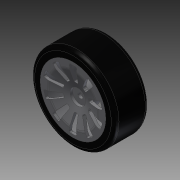
# Autodesk Inventor part: ModellingWheel_65mm
Saved by Autodesk Inventor 2014 SP1 (Build 180222100, 222)
## iProperties
Created: 2015-04-19
Part Number: ModellingWheel_65mm
Material: Rubber
Document SubType Name: Modeling
Designer: david
Density: 0.93 g/cm^3
Appearance: Rubber - Black - Version 1.1
Mass: 44.3361 g
Surface Area: 161.393 cm^2
Volume: 47.6732 cm^3
Author: david
Autodesk Inventor part; units mm, degrees
ref_plane "YZ Plane" through (0, 0, 0) normal (1, 0, 0) x (0, 1, 0)
ref_plane "XZ Plane" through (0, 0, 0) normal (0, 1, 0) x (-1, 0, 0)
ref_plane "XY Plane" through (0, 0, 0) normal (0, 0, 1) x (1, 0, 0)
sketch "Sketch1" plane through (0, 0, 0) normal (1, 0, 0) x (0, 1, 0)
  line L0 (0, 2) -> (0, 6)
  line L1 (0, 0) -> (0, -6.7762) construction
  line L2 (0, 2) -> (6.5, 2)
  line L3 (6.5, 2) -> (6.5, 9)
  line L4 (0, 0) -> (28.6637, 0) construction
  line L5 (6.5, 9) -> (0, 9)
  line L6 (0, 9) -> (-3.75, 19.25)
  line L7 (-3.75, 19.25) -> (-3.75, 23.25)
  line L8 (-3.75, 23.25) -> (20.5, 23.25)
  line L9 (20.5, 23.25) -> (20.5, 25.25)
  line L10 (20.5, 25.25) -> (-5.75, 25.25)
  line L11 (-5.75, 25.25) -> (-5.75, 19.25)
  line L12 (0, 6) -> (-2, 6)
  line L13 (-2, 6) -> (-5.75, 19.25)
  line L14 (-5.75, 19.25) -> (0.5106, 19.25) construction
  dimension "d0" = 4
  dimension "d1" = 2
  dimension "d2" = 6.5
  dimension "d3" = 9
  dimension "d4" = 23.25
  dimension "d5" = 2
  dimension "d6" = 14
  dimension "d7" = 26.25
  dimension "d8" = 2
  dimension "d9" = 2
  dimension "d10" = 6
  constraints: 30 end point, 9 perpendicular, 2 collinear, 2 parallel, 2 point on line, 1 vertical
  measures "d0" distance of L0.start L0.end
  measures "d1" distance of L1.start L0.start
  measures "d2" distance of L0.start L2.end
  measures "d3" distance from line of L4 L3.end
  measures "d4" distance between parallel lines of L4 L8
  measures "d5" distance between parallel lines of L8 L10
  measures "d6" distance between parallel lines of L9 L3
  measures "d7" distance between parallel lines of L9 L11
  measures "d8" distance between parallel lines of L11 L7
  measures "d9" distance of L0.end L12.end
  measures "d10" distance of L10.end L11.end
revolve "Revolution1" add sketch "Sketch1" angle 360 about axis through (0, 0, 0) along (0, 1, 0)
sketch "Sketch2" plane through (0, 20.5, 0) normal (0, 1, 0) x (1, 0, 0)
  circle A0 centre (0, 0) radius 25.25 projected
  circle A1 centre (0, 0) radius 32.5
  dimension "d12" = 65
  constraints: 1 centre point, 1 coincident
  measures "d12" diameter of A1
extrude "Extrusion1" add sketch "Sketch2" against normal up to surface (26.25 mm away) separate body
fillet "Fillet1" radius 3 2 edges at (-32.5, -5.75, 0) (-32.5, 20.5, 0)
sketch "Sketch3" plane through (0, 6.5, 0) normal (0, 1, 0) x (1, 0, 0)
  circle A0 centre (0, 0) radius 2 projected
  circle A1 centre (0, 0) radius 9 projected
  line L0 (6.9282, 0) -> (3.4641, -6)
  line L1 (3.4641, -6) -> (-3.4641, -6)
  line L2 (-3.4641, -6) -> (-6.9282, 0)
  line L3 (-6.9282, 0) -> (-3.4641, 6)
  line L4 (-3.4641, 6) -> (3.4641, 6)
  line L5 (3.4641, 6) -> (6.9282, 0)
  line L6 (0, 0) -> (12.5028, 0) construction
  dimension "d16" = 12
  constraints: 14 end point, 1 coincident, 1 horizontal, 1 point on line, 13 other
  measures "d16" distance between parallel lines of L0 L3
extrude "Extrusion2" cut sketch "Sketch3" against normal blind 4.5 contours L0 L1 L2 L3 L4 L5 bodies 1
sketch "Sketch4" plane through (0, -5.75, 0) normal (0, -1, 0) x (1, 0, 0)
  circle A0 centre (0, 0) radius 25.25 projected
  circle A1 centre (0, 0) radius 19.25 projected
  line L0 (-1.878, 23) -> (1.878, 23)
  line L1 (2.8714, 21.8854) -> (1.6022, 10.8854)
  line L2 (0.6087, 10) -> (-0.6087, 10)
  line L3 (-1.6022, 10.8854) -> (-2.8714, 21.8854)
  line L4 (0, 0) -> (0, 46.8233) construction
  circle A2 centre (0, 0) radius 19.25 construction
  circle A3 centre (0, 0) radius 6 construction
  circle A4 centre (0, 0) radius 25.25 construction
  circle A5 centre (0, 0) radius 19.25 construction
  circle A6 centre (0, 0) radius 19.25 construction
  circle A7 centre (0, 0) radius 25.25 construction
  circle A8 centre (0, 0) radius 29.5 construction
  circle A9 centre (0, 0) radius 25.25 construction
  arc A10 (-1.6022, 10.8854) -> (-0.6087, 10) centre (-0.6087, 11) ccw
  arc A11 (0.6087, 10) -> (1.6022, 10.8854) centre (0.6087, 11) ccw
  arc A12 (-1.878, 23) -> (-2.8714, 21.8854) centre (-1.878, 22) ccw
  arc A13 (2.8714, 21.8854) -> (1.878, 23) centre (1.878, 22) ccw
  line L5 (11.9997, 19.7112) -> (15.0384, 17.5035)
  line L6 (15.1869, 16.0179) -> (7.6944, 7.8647)
  line L7 (6.3703, 7.7324) -> (5.3854, 8.448)
  line L8 (5.1021, 9.7482) -> (10.5409, 19.3934)
  arc A14 (5.1021, 9.7482) -> (5.3854, 8.448) centre (5.9731, 9.257) ccw
  arc A15 (6.3703, 7.7324) -> (7.6944, 7.8647) centre (6.9581, 8.5414) ccw
  arc A16 (11.9997, 19.7112) -> (10.5409, 19.3934) centre (11.412, 18.9022) ccw
  arc A17 (15.1869, 16.0179) -> (15.0384, 17.5035) centre (14.4506, 16.6945) ccw
  line L9 (21.294, 8.8935) -> (22.4546, 5.3213)
  line L10 (21.7015, 4.0321) -> (10.8477, 1.84)
  line L11 (9.6987, 2.5112) -> (9.3225, 3.6691)
  line L12 (9.8575, 4.8875) -> (19.9269, 9.4938)
  arc A18 (9.8575, 4.8875) -> (9.3225, 3.6691) centre (10.2735, 3.9781) ccw
  arc A19 (9.6987, 2.5112) -> (10.8477, 1.84) centre (10.6497, 2.8202) ccw
  arc A20 (21.294, 8.8935) -> (19.9269, 9.4938) centre (20.3429, 8.5844) ccw
  arc A21 (21.7015, 4.0321) -> (22.4546, 5.3213) centre (21.5036, 5.0123) ccw
  line L13 (22.4546, -5.3213) -> (21.294, -8.8935)
  line L14 (19.9269, -9.4938) -> (9.8575, -4.8875)
  line L15 (9.3225, -3.6691) -> (9.6987, -2.5112)
  line L16 (10.8477, -1.84) -> (21.7015, -4.0321)
  arc A22 (10.8477, -1.84) -> (9.6987, -2.5112) centre (10.6497, -2.8202) ccw
  arc A23 (9.3225, -3.6691) -> (9.8575, -4.8875) centre (10.2735, -3.9781) ccw
  arc A24 (22.4546, -5.3213) -> (21.7015, -4.0321) centre (21.5036, -5.0123) ccw
  arc A25 (19.9269, -9.4938) -> (21.294, -8.8935) centre (20.3429, -8.5844) ccw
  line L17 (15.0384, -17.5035) -> (11.9997, -19.7112)
  line L18 (10.5409, -19.3934) -> (5.1021, -9.7482)
  line L19 (5.3854, -8.448) -> (6.3703, -7.7324)
  line L20 (7.6944, -7.8647) -> (15.1869, -16.0179)
  arc A26 (7.6944, -7.8647) -> (6.3703, -7.7324) centre (6.9581, -8.5414) ccw
  arc A27 (5.3854, -8.448) -> (5.1021, -9.7482) centre (5.9731, -9.257) ccw
  arc A28 (15.0384, -17.5035) -> (15.1869, -16.0179) centre (14.4506, -16.6945) ccw
  arc A29 (10.5409, -19.3934) -> (11.9997, -19.7112) centre (11.412, -18.9022) ccw
  line L21 (1.878, -23) -> (-1.878, -23)
  line L22 (-2.8714, -21.8854) -> (-1.6022, -10.8854)
  line L23 (-0.6087, -10) -> (0.6087, -10)
  line L24 (1.6022, -10.8854) -> (2.8714, -21.8854)
  arc A30 (1.6022, -10.8854) -> (0.6087, -10) centre (0.6087, -11) ccw
  arc A31 (-0.6087, -10) -> (-1.6022, -10.8854) centre (-0.6087, -11) ccw
  arc A32 (1.878, -23) -> (2.8714, -21.8854) centre (1.878, -22) ccw
  arc A33 (-2.8714, -21.8854) -> (-1.878, -23) centre (-1.878, -22) ccw
  line L25 (-11.9997, -19.7112) -> (-15.0384, -17.5035)
  line L26 (-15.1869, -16.0179) -> (-7.6944, -7.8647)
  line L27 (-6.3703, -7.7324) -> (-5.3854, -8.448)
  line L28 (-5.1021, -9.7482) -> (-10.5409, -19.3934)
  arc A34 (-5.1021, -9.7482) -> (-5.3854, -8.448) centre (-5.9731, -9.257) ccw
  arc A35 (-6.3703, -7.7324) -> (-7.6944, -7.8647) centre (-6.9581, -8.5414) ccw
  arc A36 (-11.9997, -19.7112) -> (-10.5409, -19.3934) centre (-11.412, -18.9022) ccw
  arc A37 (-15.1869, -16.0179) -> (-15.0384, -17.5035) centre (-14.4506, -16.6945) ccw
  line L29 (-21.294, -8.8935) -> (-22.4546, -5.3213)
  line L30 (-21.7015, -4.0321) -> (-10.8477, -1.84)
  line L31 (-9.6987, -2.5112) -> (-9.3225, -3.6691)
  line L32 (-9.8575, -4.8875) -> (-19.9269, -9.4938)
  arc A38 (-9.8575, -4.8875) -> (-9.3225, -3.6691) centre (-10.2735, -3.9781) ccw
  arc A39 (-9.6987, -2.5112) -> (-10.8477, -1.84) centre (-10.6497, -2.8202) ccw
  arc A40 (-21.294, -8.8935) -> (-19.9269, -9.4938) centre (-20.3429, -8.5844) ccw
  arc A41 (-21.7015, -4.0321) -> (-22.4546, -5.3213) centre (-21.5036, -5.0123) ccw
  line L33 (-22.4546, 5.3213) -> (-21.294, 8.8935)
  line L34 (-19.9269, 9.4938) -> (-9.8575, 4.8875)
  line L35 (-9.3225, 3.6691) -> (-9.6987, 2.5112)
  line L36 (-10.8477, 1.84) -> (-21.7015, 4.0321)
  arc A42 (-10.8477, 1.84) -> (-9.6987, 2.5112) centre (-10.6497, 2.8202) ccw
  arc A43 (-9.3225, 3.6691) -> (-9.8575, 4.8875) centre (-10.2735, 3.9781) ccw
  arc A44 (-22.4546, 5.3213) -> (-21.7015, 4.0321) centre (-21.5036, 5.0123) ccw
  arc A45 (-19.9269, 9.4938) -> (-21.294, 8.8935) centre (-20.3429, 8.5844) ccw
  line L37 (-15.0384, 17.5035) -> (-11.9997, 19.7112)
  line L38 (-10.5409, 19.3934) -> (-5.1021, 9.7482)
  line L39 (-5.3854, 8.448) -> (-6.3703, 7.7324)
  line L40 (-7.6944, 7.8647) -> (-15.1869, 16.0179)
  arc A46 (-7.6944, 7.8647) -> (-6.3703, 7.7324) centre (-6.9581, 8.5414) ccw
  arc A47 (-5.3854, 8.448) -> (-5.1021, 9.7482) centre (-5.9731, 9.257) ccw
  arc A48 (-15.0384, 17.5035) -> (-15.1869, 16.0179) centre (-14.4506, 16.6945) ccw
  arc A49 (-10.5409, 19.3934) -> (-11.9997, 19.7112) centre (-11.412, 18.9022) ccw
  point P0 (-3, 23)
  point P1 (3, 23)
  point P2 (1.5, 10)
  point P3 (-1.5, 10)
  point P4 (11.092, 20.3707)
  point P5 (15.9461, 16.844)
  point P6 (7.0914, 7.2085)
  point P7 (4.6643, 8.9718)
  point P8 (20.9472, 9.9606)
  point P9 (22.8014, 4.2542)
  point P10 (9.9741, 1.6636)
  point P11 (9.047, 4.5168)
  point P12 (22.8014, -4.2542)
  point P13 (20.9472, -9.9606)
  point P14 (9.047, -4.5168)
  point P15 (9.9741, -1.6636)
  point P16 (15.9461, -16.844)
  point P17 (11.092, -20.3707)
  point P18 (4.6643, -8.9718)
  point P19 (7.0914, -7.2085)
  point P20 (3, -23)
  point P21 (-3, -23)
  point P22 (-1.5, -10)
  point P23 (1.5, -10)
  point P24 (-11.092, -20.3707)
  point P25 (-15.9461, -16.844)
  point P26 (-7.0914, -7.2085)
  point P27 (-4.6643, -8.9718)
  point P28 (-20.9472, -9.9606)
  point P29 (-22.8014, -4.2542)
  point P30 (-9.9741, -1.6636)
  point P31 (-9.047, -4.5168)
  point P32 (-22.8014, 4.2542)
  point P33 (-20.9472, 9.9606)
  point P34 (-9.047, 4.5168)
  point P35 (-9.9741, 1.6636)
  point P36 (-15.9461, 16.844)
  point P37 (-11.092, 20.3707)
  point P38 (-4.6643, 8.9718)
  point P39 (-7.0914, 7.2085)
  dimension "d19" = 13
  dimension "d20" = 6
  dimension "d21" = 3
  dimension "d22" = 10
  dimension "d23" = 1
  dimension "d24" = 1
  dimension "d27" = 360
  constraints: 82 end point, 80 point on circle, 80 point on line, 40 centre point, 8 tangent, 2 equal radius, 1 horizontal, 1 parallel, 1 perpendicular, 242 other
  measures "d19" distance between parallel lines of L2 L0
  measures "d20" distance of point (-3, 23) point (3, 23)
  measures "d21" distance of point (1.5, 10) point (-1.5, 10)
  measures "d22" distance from line of A0.centre L2
  measures "d23" radius of A10
  measures "d24" radius of A13
extrude "Extrusion3" cut sketch "Sketch4" against normal through all contours L10 A19 L11 A18 L12 A1 | A1 L12 A20 L9 A21 L10 | L16 A24 L13 A25 L14 A1 | A1 L14 A23 L15 A22 L16 | L6 A15 L7 A14 L8 A1 | A1 L8 A16 L5 A17 L6 | L20 A28 L17 A29 L18 A1 | A1 L18 A27 L19 A26 L20 | L1 A11 L2 A10 L3 A1 | A1 L3 A12 L0 A13 L1 | L24 A32 L21 A33 L22 A1 | A1 L22 A31 L23 A30 L24 | L38 A47 L39 A46 L40 A1 | A1 L40 A48 L37 A49 L38 | L28 A36 L25 A37 L26 A1 | A1 L26 A35 L27 A34 L28 | L34 A43 L35 A42 L36 A1 | A1 L36 A44 L33 A45 L34 | L32 A40 L29 A41 L30 A1 | A1 L30 A39 L31 A38 L32 bodies 1
fillet "Fillet2" radius 5 10 edges at (15.5736, -5.75, -11.3149) (19.25, -5.75, 0) (5.9486, -5.75, -18.3078) (-5.9486, -5.75, -18.3078) (15.5736, -5.75, 11.3149) (-15.5736, -5.75, -11.3149) (-19.25, -5.75, 0) (-15.5736, -5.75, 11.3149) (-5.9486, -5.75, 18.3078) (5.9486, -5.75, 18.3078)
fillet "Fillet2" radius 5 10 edges at (15.5736, -3.75, -11.3149) (19.25, -3.75, 0) (15.5736, -3.75, 11.3149) (5.9486, -3.75, 18.3078) (-5.9486, -3.75, 18.3078) (-15.5736, -3.75, 11.3149) (-19.25, -3.75, 0) (-15.5736, -3.75, -11.3149) (-5.9486, -3.75, -18.3078) (5.9486, -3.75, -18.3078)
body "Solid1"
body "Solid2"
